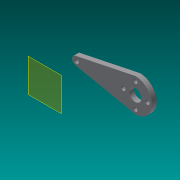
# Autodesk Inventor part: headtilt-teardrop
Saved by Autodesk Inventor 2013 SP2 (Build 170200200, 200)
## iProperties
Created: 2014-11-25
Part Number: headtilt-teardrop
Material: Generic
Document SubType Name: Sheet Metal
Designer: Master
Density: 1 g/cm^3
Sheet Metal Rule: Default
Author: Master
Autodesk Inventor part; units mm, degrees
ref_plane "YZ Plane" through (0, 0, 0) normal (1, 0, 0) x (0, 1, 0)
ref_plane "XZ Plane" through (0, 0, 0) normal (0, 1, 0) x (-1, 0, 0)
ref_plane "XY Plane" through (0, 0, 0) normal (0, 0, 1) x (1, 0, 0)
sketch "Sketch1" plane through (0, 0, 0) normal (0, 0, 1) x (1, 0, 0)
  line L0 (53.6991, 27.6003) -> (52.1809, 27.6003)
  arc A0 (53.6991, 27.1003) -> (53.6991, 27.6003) centre (55.1781, 27.3503) ccw
  line L1 (52.1809, 27.1003) -> (53.6991, 27.1003)
  arc A1 (52.1809, 27.1003) -> (52.1809, 27.6003) centre (63.1781, 27.3503) ccw
  circle A2 centre (63.1781, 35.3503) radius 1.5
  circle A3 centre (63.1781, 19.3503) radius 1.5
  circle A4 centre (71.1781, 27.3503) radius 1.5
  circle A5 centre (63.1781, 27.3503) radius 4
  circle A6 centre (24.1779, 27.3503) radius 1.4986
  arc A7 (24.1777, 30.2419) -> (24.1781, 24.4588) centre (24.1779, 27.3503) ccw
  line L2 (24.1777, 30.2419) -> (63.1781, 38.3503)
  line L3 (24.1781, 24.4588) -> (63.1794, 16.3503)
  arc A8 (63.1794, 16.3503) -> (63.1781, 38.3503) centre (63.1781, 27.3503) ccw
  circle A9 centre (63.1781, 35.3503) radius 1.5
  arc A10 (53.6991, 27.1003) -> (53.6991, 27.6003) centre (55.1781, 27.3503) ccw
  circle A11 centre (63.1781, 19.3503) radius 1.5
  circle A12 centre (71.1781, 27.3503) radius 1.5
  circle A13 centre (55.1781, 27.3503) radius 1.5
  circle A14 centre (63.1781, 35.3503) radius 1.5
  circle A15 centre (63.1781, 19.3503) radius 1.5
  circle A16 centre (71.1781, 27.3503) radius 1.5
  circle A17 centre (63.1781, 27.3503) radius 1.75
  circle A18 centre (63.1781, 27.3503) radius 1.75
  point P0 (0, 0)
  dimension "d1" = 2.9972
  measures "d1" diameter of A6
extrude "Plate1" add sketch "Sketch1" along normal blind 3.175 contours A13 L1 A1 L3 A7 L2 L0 | L0 A1 L2 L3 L1 A0
sketch "Sketch2" plane through (0, 0, 0) normal (0, 0, -1) x (-1, 0, 0)
  arc A0 (-63.1781, 38.3503) -> (-63.1794, 16.3503) centre (-63.1781, 27.3503) ccw
  line L0 (-24.1781, 24.4588) -> (-63.1794, 16.3503)
  arc A1 (-24.1781, 24.4588) -> (-24.1777, 30.2419) centre (-24.1779, 27.3503) ccw
  line L1 (-63.1781, 38.3503) -> (-24.1777, 30.2419)
  arc A2 (-23.923, 22.285) -> (-23.9226, 32.4157) centre (-24.1779, 27.3503) ccw
  line L2 (-23.923, 22.285) -> (-62.9453, 14.1721)
  arc A3 (-62.9438, 40.5285) -> (-62.9453, 14.1721) centre (-63.1781, 27.3503) ccw
  line L3 (-62.9438, 40.5285) -> (-23.9226, 32.4157)
  point P0 (0, 0)
sheet face with bend "Face2" sketch "Sketch2" thickness 3.175 toward (0, 0, 1) bend radius 3.175 relief straight relief width 3.175 relief depth 1.5875
bend "Bend1"
sketch "Sketch3" plane through (0, 0, 3.175) normal (0, 0, 1) x (1, 0, 0)
  circle A0 centre (71.1781, 27.3503) radius 1.5
  circle A1 centre (63.1781, 19.3503) radius 1.5
  circle A2 centre (63.1781, 35.3503) radius 1.5
  circle A3 centre (55.1781, 27.3503) radius 1.5
  circle A4 centre (63.1781, 35.3503) radius 1
  circle A5 centre (55.1781, 27.3503) radius 1
  circle A6 centre (63.1781, 19.3503) radius 1
  circle A7 centre (71.1781, 27.3503) radius 1
  point P0 (0, 0)
  dimension "d8" = 2
  dimension "d9" = 2
  dimension "d10" = 2
  dimension "d11" = 2
  measures "d8" diameter of A4
  measures "d9" diameter of A5
  measures "d10" diameter of A6
  measures "d11" diameter of A7
sheet face with bend "Face3" sketch "Sketch3" thickness 3.175 toward (0, 0, -1) bend radius 3.175 relief straight relief width 3.175 relief depth 1.5875
bend "Bend2"
ref_plane "Work Plane2" through (0, 0, 0) normal (0, 0, 1) x (1, 0, 0)
sketch "Sketch4" plane through (0, 0, 3.175) normal (0, 0, 1) x (1, 0, 0)
  circle A0 centre (63.1781, 35.3503) radius 1 projected
  circle A1 centre (71.1781, 27.3503) radius 1 projected
  circle A2 centre (63.1781, 19.3503) radius 1 projected
  circle A3 centre (55.1781, 27.3503) radius 1 projected
  line L0 (23.9226, 32.4157) -> (62.9438, 40.5285) projected
  arc A4 (23.9226, 32.4157) -> (23.923, 22.285) centre (24.1779, 27.3503) ccw projected
  line L1 (62.9453, 14.1721) -> (23.923, 22.285) projected
  arc A5 (62.9453, 14.1721) -> (62.9438, 40.5285) centre (63.1781, 27.3503) ccw projected
  circle A6 centre (63.1781, 27.3503) radius 4 projected
  circle A7 centre (24.1779, 27.3503) radius 1.4986 projected
  circle A8 centre (24.1779, 27.3503) radius 1
  point P0 (0, 0)
  dimension "d17" = 2
  constraints: 1 centre point, 1 coincident
  measures "d17" diameter of A8
equation "\"d3\" = BendRadius"
equation "\"d4\" = BendReliefWidth"
equation "\"d6\" = MinimumRemnant"
equation "\"d5\" = BendReliefDepth"
equation "\"d7\" = BendRadius"
equation "\"d12\" = BendRadius"
equation "\"d13\" = BendReliefWidth"
equation "\"d15\" = MinimumRemnant"
equation "\"d14\" = BendReliefDepth"
equation "\"d16\" = BendRadius"
equation "\"BendRadius\" = Thickness"
equation "\"BendReliefWidth\" = Thickness"
equation "\"BendReliefDepth\" = 0.5 * Thickness"
equation "\"CornerReliefSize\" = 4 * Thickness"
equation "\"MinimumRemnant\" = 2 * Thickness"
equation "\"TransitionRadius\" = BendRadius"
equation "\"JacobiRadiusSize\" = BendRadius"
equation "\"GapSize\" = Thickness"
equation "\"d2\" = BendRadius"
equation "\"Thickness\" = 3.175"
body "Solid1"
